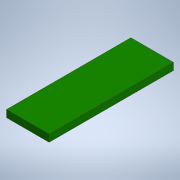
# Autodesk Inventor part: akkum_board2
Saved by Autodesk Inventor 2022 (Build 260153000, 153)
## iProperties
Created: 2022-12-04
Part Number: akkum_board2
Material: Generic
Document SubType Name: Modeling
Designer: akapu
Density: 1 g/cm^3
Appearance: Default
Author: akapu
Autodesk Inventor part; units mm, degrees
ref_plane "YZ Plane" through (0, 0, 0) normal (1, 0, 0) x (0, 1, 0)
ref_plane "XZ Plane" through (0, 0, 0) normal (0, 1, 0) x (-1, 0, 0)
ref_plane "XY Plane" through (0, 0, 0) normal (0, 0, 1) x (1, 0, 0)
sketch "Sketch1" plane through (0, 0, 0) normal (0, 1, 0) x (-1, 0, 0)
  line L0 (0, 0) -> (-20.1, 0)
  line L1 (-20.1, 0) -> (-20.1, -58.7)
  line L2 (-20.1, -58.7) -> (0, -58.7)
  line L3 (0, -58.7) -> (0, 0)
  dimension "d0" = 20.1
  dimension "d1" = 58.7
  constraints: 8 end point, 2 parallel, 1 horizontal, 1 perpendicular
  measures "d0" distance of L2.end L1.end
  measures "d1" distance of L1.end L0.end
extrude "Extrusion1" add sketch "Sketch1" along normal blind 3.4
body "Solid1"
